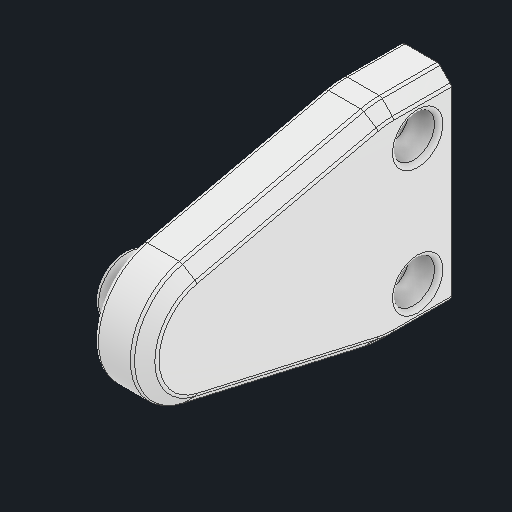
# Autodesk Inventor part: 롤축지지대베어링
Saved by Autodesk Inventor 2027.1 (Build 311270010, 270A)
## iProperties
Created: 2026-08-11
Part Number: 롤축지지대베어링
Material: ABS 플라스틱
Document SubType Name: Modeling
Designer: moieboy9999
Density: 1.06 g/cm^3
Appearance: 매끄러움 - 흰색
Mass: 4.42901 g
Surface Area: 21.6177 cm^2
Volume: 4.17831 cm^3
Author: moieboy9999
## iProperties of the stored document 롤축지지대베어링_3D 인쇄.ipt
Created: 2026-08-14
Part Number: 롤축지지대베어링_3D 인쇄
Material: 일반
Document SubType Name: Modeling
Designer: maker
Density: 1 g/cm^3
Appearance: 기본값
Author: maker
Autodesk Inventor part; units mm, degrees
ref_plane "YZ Plane" through (0, 0, 0) normal (1, 0, 0) x (0, 1, 0)
ref_plane "XZ Plane" through (0, 0, 0) normal (0, 1, 0) x (-1, 0, 0)
ref_plane "XY Plane" through (0, 0, 0) normal (0, 0, 1) x (1, 0, 0)
sketch "스케치1" plane through (0, 0, 0) normal (1, 0, 0) x (0, 1, 0)
  circle A0 centre (0, 0) radius 1.5
  circle A1 centre (0, 0) radius 2.5
  line L0 (0, 0) -> (0, -4)
  line L1 (0, -4) -> (5, -4)
  line L2 (5, -4) -> (-20, -4)
  line L3 (-20, -4) -> (-20, 4)
  line L4 (-20, 4) -> (5, 4)
  line L5 (5, 4) -> (5, -4)
  circle A2 centre (-15, 0) radius 1.5
  circle A3 centre (-15, 0) radius 2.5
  line L6 (-15, 0) -> (-15, 25)
  line L7 (-15, 25) -> (-7.5, 25)
  circle A4 centre (-7.5, 25) radius 3.5
  circle A5 centre (-7.5, 25) radius 7.5
  line L8 (5, 4) -> (-0.189, 26.6732)
  line L9 (-20, 4) -> (-14.811, 26.6732)
  point P0 (-14.811, 26.6732)
  dimension "d0" = 3
  dimension "d1" = 5
  dimension "d2" = 4
  dimension "d3" = 5
  dimension "d4" = 25
  dimension "d5" = 8
  dimension "d8" = 15
  dimension "d13" = 25
  dimension "d14" = 7.5
  dimension "d15" = 7
  dimension "d16" = 15
  constraints: 20 end point, 6 centre point, 5 coincident, 3 horizontal, 2 parallel, 2 perpendicular, 2 point on circle, 2 tangent, 2 vertical, 4 other
  measures "d0" diameter of A0
  measures "d1" diameter of A1
  measures "d2" distance of L0.start L0.end
  measures "d3" distance of L0.end L1.end
  measures "d4" distance of L3.end L4.end
  measures "d5" distance of L2.end L3.end
  measures "d8" distance of A0.centre A2.centre
  measures "d13" distance of L6.start L6.end
  measures "d14" distance of L6.end L7.end
  measures "d15" diameter of A4
  measures "d16" diameter of A5
extrude "돌출1" add sketch "스케치1" along normal blind 4 contours L2 L3 L4 L5 L1 | L4 L6 A5 L8 | L9 A5 L6 L4 | A5
extrude "돌출2" add sketch "스케치1" along normal blind 2 contours A1 | A3
sketch "스케치2" plane through (4, 0, 0) normal (1, 0, 0) x (0, 0, -1)
  circle A0 centre (-25, -7.5) radius 3.5 projected
  circle A1 centre (-25, -7.5) radius 3.5
  point P0 (0, 0)
  constraints: 1 centre point, 1 coincident
extrude "돌출3" add sketch "스케치2" against normal blind 8
move faces "이동2" translate (2, 0, 0) faces at (4, -5.2955, 18.5613)
fillet "모깎기1" radius 2 1 edges at (0, -7.5, 28.5)
fillet "모깎기2" radius 10 2 edges at (3, 5, 4) (3, -20, 4)
chamfer "모따기1" distance 1.5 angle 45 7 edges at (6, -17.2795, 15.8872) (6, -19.9368, 3.9929) (6, -20, -0.5649) (6, -7.5, 32.5) (6, 2.2795, 15.8872) (6, 4.9368, 3.9929) (6, 5, -0.5649)
fillet "모깎기3" radius 0.5 14 edges at (6, -7.5, 31) (6, 0.8173, 15.5526) (6, 3.4463, 3.8245) (6, 3.5, -0.5649) (6, -18.4463, 3.8245) (6, -18.5, -0.5649) (6, -15.8173, 15.5526) (4.5, -19.9368, 3.9929) (4.5, -20, -0.5649) (4.5, -7.5, 32.5) (4.5, 2.2795, 15.8872) (4.5, 4.9368, 3.9929) (4.5, 5, -0.5649) (4.5, -17.2795, 15.8872)
fillet "모깎기4" radius 0.5 7 edges at (0, -19.9368, 3.9929) (0, -17.2795, 15.8872) (0, -7.5, 32.5) (0, 2.2795, 15.8872) (0, 4.9368, 3.9929) (0, 5, -0.5649) (0, -20, -0.5649)
fillet "모깎기5" radius 0.5 1 edges at (-4, -7.5, 28.5)
move faces "이동1" translate (0.5, 0, 0) faces at (2, -12.8575, 0.1994) (2, 2.1279, 0.3191)
fillet "모깎기6" radius 0.5 2 edges at (6, -2.5, 0) (6, -17.5, 0)
